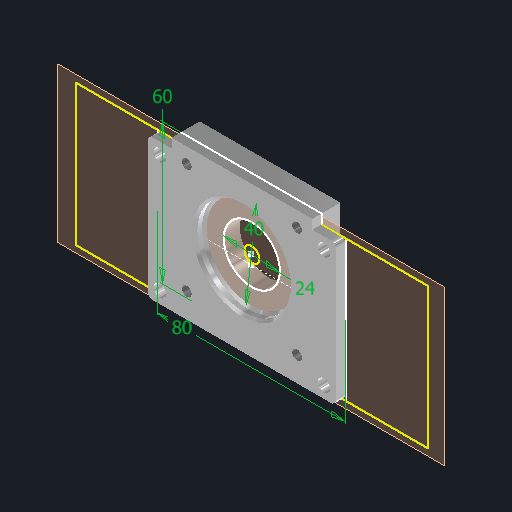
# Autodesk Inventor part: Montura de Motor
Saved by Autodesk Inventor 2022 (Build 260153000, 153)
## iProperties
Created: 2021-09-13
Part Number: Montura de Motor
Material: Aluminum 6061
Document SubType Name: Modeling
Designer: Andres
Density: 2.7 g/cm^3
Appearance: Aluminum - Flat
Author: Andres
Autodesk Inventor part; units mm, degrees
ref_plane "YZ Plane" through (0, 0, 0) normal (1, 0, 0) x (0, 1, 0)
ref_plane "XZ Plane" through (0, 0, 0) normal (0, 1, 0) x (-1, 0, 0)
ref_plane "XY Plane" through (0, 0, 0) normal (0, 0, 1) x (1, 0, 0)
ref_plane "Work Plane1" through (0, 0, 0) normal (0, 0, 1) x (1, 0, 0)
sketch "Sketch1" plane through (0, 0, 0) normal (0, 0, 1) x (1, 0, 0)
  line L0 (45, 9) -> (45, 60) projected
  line L1 (0, 60) -> (45, 60) projected
  line L2 (0, 0) -> (0, 60) projected
  line L3 (0, 0) -> (150, 0) projected
  line L4 (150, 0) -> (150, 60) projected
  line L5 (105, 60) -> (150, 60) projected
  line L6 (105, 60) -> (105, 9) projected
  arc A0 (100, 4) -> (105, 9) centre (100, 9) ccw projected
  line L7 (100, 4) -> (50, 4) projected
  arc A1 (45, 9) -> (50, 4) centre (50, 9) ccw projected
  circle A2 centre (51.5, 57.5) radius 2.5 projected
  circle A3 centre (98.5, 57.5) radius 2.5 projected
  circle A4 centre (98.5, 10.5) radius 2.5 projected
  circle A5 centre (51.5, 10.5) radius 2.5 projected
  line L8 (35, 60) -> (35, 0)
  line L9 (115, 60) -> (115, 0)
  line L10 (115, 30) -> (35, 30) construction
  circle A6 centre (75, 34) radius 3.175 projected
  circle A7 centre (75, 34) radius 20
  line L11 (45, 60) -> (45, 64)
  line L12 (45, 64) -> (105, 64)
  line L13 (105, 64) -> (105, 60)
  circle A8 centre (75, 34) radius 12
  point P0 (75, 30)
  dimension "d0" = 40
  dimension "d1" = 80
  dimension "d4" = 60
  dimension "d28" = 24
  constraints: 12 end point, 4 point on line, 3 midpoint, 2 centre point, 2 coincident, 2 perpendicular, 2 vertical, 1 horizontal, 1 vertical alignment
  measures "d0" diameter of A7
  measures "d1" distance of L10.start L10.end
  measures "d4" distance between parallel lines of L7 L12
  measures "d28" diameter of A8
extrude "Extrusion1" add sketch "Sketch1" along normal blind 4 contours A1 L7 A0 L6 L5 L9 L3 L8 L1 L0 | L0 L11 L12 L13 L6 A0 L7 A1 | A2 | A3 | A4 | A5
ref_plane "Work Plane2" through (45, 4, -8) normal (0, 0, 1) x (1, 0, 0)
extrude "Extrusion2" add sketch "Sketch1" against normal up to surface (8 mm away) contours L0 L11 L12 L13 L6 A0 L7 A1 | A2 | A3 | A4 | A5 | A7
sketch "Sketch2" plane through (0, 0, 4) normal (0, 0, 1) x (1, 0, 0)
  circle A0 centre (51.5, 57.5) radius 2.5 projected
  circle A1 centre (98.5, 57.5) radius 2.5 projected
  circle A2 centre (98.5, 10.5) radius 2.5 projected
  circle A3 centre (51.5, 10.5) radius 2.5 projected
  point P0 (0, 0)
hole "Hole1" at (51.5, 57.5, 4) at (51.5, 10.5, 4) at (98.5, 10.5, 4) at (98.5, 57.5, 4) direction (0, 0, -1) diameter 4.134 depth 10 tip angle 118 thread size "M5x0.8" class "6H" standard "ISO Metric profile"
sketch "Sketch3" plane through (0, 0, 4) normal (0, 0, 1) x (1, 0, 0)
  line L0 (40, 55) -> (110, 55) construction
  line L1 (110, 55) -> (110, 5) construction
  line L2 (110, 5) -> (40, 5) construction
  line L3 (40, 5) -> (40, 55) construction
  line L4 (40, 55) -> (110, 5) construction
  line L5 (110, 55) -> (40, 5) construction
  circle A0 centre (75, 34) radius 20 projected
  point P0 (0, 0)
  point P1 (75, 30)
  dimension "d14" = 70
  dimension "d15" = 50
  dimension "d23" = 4
  constraints: 12 end point, 4 coincident, 2 parallel, 1 horizontal, 1 midpoint, 1 perpendicular, 1 vertical alignment
  measures "d14" distance of L1.end L2.end
  measures "d15" distance of L0.end L1.end
  measures "d23" distance of point (75, 30) A0.centre
hole "Hole2" at (40, 55, 4) at (40, 5, 4) at (110, 5, 4) at (110, 55, 4) direction (0, 0, -1) diameter 5.3 depth 4 tip angle 118 clearance for "Countersunk Flat Head Screw ISO 2009/7046" size "M5" standard "ISO"
fillet "Fillet1" radius 2 4 edges at (35, 60, 2) (35, 0, 2) (115, 0, 2) (115, 60, 2)
chamfer "Chamfer1" distance 1 angle 45 1 edges at (55, 34, 4)
chamfer "Chamfer2" distance 1 angle 45 1 edges at (55, 34, 0)
chamfer "Chamfer3" distance 1 angle 45 1 edges at (63, 34, -8)
body "Solid1"
